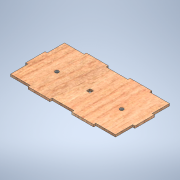
# Autodesk Inventor part: TAPA4
Saved by Autodesk Inventor 2021 (Build 250183000, 183)
## iProperties
Created: 2019-12-05
Part Number: TAPA4
Material: Generic
Document SubType Name: Modeling
Designer: Carlos Loaiza
Density: 1 g/cm^3
Appearance: Default
Author: Carlos Loaiza
Autodesk Inventor part; units mm, degrees
ref_plane "YZ Plane" through (0, 0, 0) normal (1, 0, 0) x (0, 1, 0)
ref_plane "XZ Plane" through (0, 0, 0) normal (0, 1, 0) x (-1, 0, 0)
ref_plane "XY Plane" through (0, 0, 0) normal (0, 0, 1) x (1, 0, 0)
sketch "Sketch1" plane through (0, 0, 0) normal (0, 0, 1) x (1, 0, 0)
  line L0 (0, 0) -> (150, 0)
  line L1 (150, 0) -> (150, 80)
  line L2 (150, 80) -> (0, 80)
  line L3 (0, 80) -> (0, 0)
  dimension "d0" = 150
  dimension "d1" = 80
  constraints: 8 end point, 3 perpendicular, 1 horizontal
  measures "d0" distance of L0.start L0.end
  measures "d1" distance of L0.end L1.end
extrude "Extrusion1" add sketch "Sketch1" along normal blind 3
sketch "Sketch2" plane through (0, 0, 3) normal (0, 0, 1) x (1, 0, 0)
  line L0 (0, 80) -> (0, 0)
  line L1 (150, 0) -> (150, 80)
  line L2 (3, 80) -> (3, 53.3333)
  line L3 (3, 53.3333) -> (0, 53.3333)
  line L4 (0, 53.3333) -> (0, 26.6667)
  line L5 (0, 26.6667) -> (3, 26.6667)
  line L6 (3, 26.6667) -> (3, 0)
  line L7 (0, 80) -> (0, 53.3333)
  line L8 (0, 26.6667) -> (0, 0)
  line L9 (147, 80) -> (147, 53.3333)
  line L10 (147, 53.3333) -> (150, 53.3333)
  line L11 (150, 53.3333) -> (150, 26.6667)
  line L12 (150, 26.6667) -> (147, 26.6667)
  line L13 (147, 26.6667) -> (147, 0)
  line L14 (150, 0) -> (150, 26.6667)
  line L15 (150, 53.3333) -> (150, 80)
  line L16 (0, 26.6667) -> (0, 0)
  line L17 (0, 0) -> (0, 3)
  line L18 (0, 3) -> (30, 3)
  line L19 (30, 3) -> (30, 0)
  line L20 (30, 0) -> (60, 0)
  line L21 (0, 0) -> (150, 0)
  line L22 (60, 0) -> (60, 3)
  line L23 (60, 3) -> (90, 3)
  line L24 (90, 3) -> (90, 0)
  line L25 (90, 0) -> (120, 0)
  line L26 (120, 0) -> (120, 3)
  line L27 (120, 3) -> (150, 3)
  line L28 (0, 80) -> (0, 77)
  line L29 (0, 77) -> (30, 77)
  line L30 (30, 77) -> (30, 80)
  line L31 (60, 80) -> (60, 77)
  line L32 (30, 80) -> (60, 80)
  line L33 (0, 80) -> (150, 80)
  line L34 (60, 77) -> (90, 77)
  line L35 (90, 77) -> (90, 80)
  line L36 (120, 80) -> (120, 77)
  line L37 (120, 77) -> (150, 77)
  line L38 (90, 80) -> (120, 80)
  line L39 (0, 0) -> (30, 0)
  line L40 (0, 0) -> (150, 0) projected
  line L41 (120, 0) -> (150, 0)
  line L42 (150, 0) -> (150, 80) projected
  line L43 (150, 80) -> (120, 80)
  line L44 (150, 80) -> (0, 80) projected
  line L45 (30, 80) -> (0, 80)
  dimension "d4" = 3
  dimension "d5" = 26.6667
  dimension "d6" = 26.6667
  dimension "d7" = 3
  dimension "d8" = 26.6667
  dimension "d9" = 26.6667
  dimension "d10" = 3
  dimension "d11" = 30
  dimension "d12" = 30
  dimension "d13" = 30
  dimension "d14" = 30
  constraints: 86 end point, 24 point on line, 9 perpendicular, 5 collinear, 3 parallel, 1 horizontal, 1 vertical, 1 other
  measures "d4" distance of L33.start L2.start
  measures "d5" distance of L2.start L3.start
  measures "d6" distance of L3.end L8.start
  measures "d7" distance of L33.end L9.start
  measures "d8" distance of L9.start L10.start
  measures "d9" distance of L11.start L14.end
  measures "d10" distance of L21.start L18.start
  measures "d11" distance of L18.start L19.start
  measures "d12" distance of L20.start L20.end
  measures "d13" distance of L22.end L23.end
  measures "d14" distance of L25.start L25.end
extrude "Extrusion2" cut sketch "Sketch2" against normal blind 3 contours L33 L2 L29 L0 | L29 L2 L3 L0 | L33 L30 L29 L2 | L5 L6 L18 L0 | L33 L35 L34 L31 | L18 L6 L21 L0 | L18 L19 L21 L6 | L33 L9 L37 L36 | L33 L1 L37 L9 | L37 L1 L10 L9 | L22 L23 L24 L21 | L26 L27 L13 L21 | L1 L27 L13 L12 | L13 L27 L1 L21
sketch "Sketch3" plane through (0, 0, 3) normal (0, 0, 1) x (1, 0, 0)
  line L0 (60, 77) -> (90, 77) projected
  line L1 (90, 3) -> (60, 3) projected
  line L2 (0, 53.3333) -> (0, 26.6667) projected
  line L3 (150, 26.6667) -> (150, 53.3333) projected
  line L4 (80, 40) -> (80, 35)
  line L5 (80, 35) -> (75, 35)
  line L6 (75, 35) -> (75, 40)
  line L7 (75, 40) -> (80, 40)
  circle A0 centre (32.0086, 37.5) radius 2.5
  circle A1 centre (120.9557, 37.5) radius 2.5
  point P0 (0, 0)
  dimension "d22" = 5
  dimension "d23" = 5
  dimension "d24" = 5
  dimension "d25" = 5
  constraints: 8 end point, 2 centre point, 2 horizontal, 1 perpendicular
  measures "d22" distance of L4.start L4.end
  measures "d23" distance of L4.end L5.end
  measures "d24" diameter of A0
  measures "d25" diameter of A1
extrude "Extrusion3" cut sketch "Sketch3" against normal blind 3
body "Solid1"
